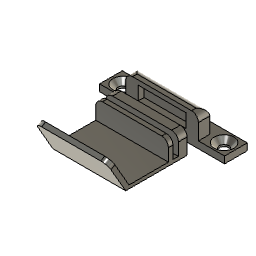
Door_Handle (Autodesk Fusion 360 design; units mm, degrees)
Autodesk Fusion 360 part; units mm, degrees
sketch "Sketch1" plane through (0, 0, 0) normal (0, 0, 1) x (1, 0, 0) in component "Door Handle"
  line L0 (16.0106, 11.1087) -> (16.0106, 8.7087)
  line L1 (-15.9894, -12.0913) -> (-15.9894, 14.9087)
  line L2 (16.0106, 8.7087) -> (16.0106, 6.7087)
  line L3 (-15.9894, 14.9087) -> (16.0106, 14.9087)
  line L4 (16.0106, 8.7087) -> (-15.9894, 8.7087)
  line L5 (16.0106, 14.9087) -> (16.0106, 11.1087)
  line L6 (16.0106, -12.0913) -> (-15.9894, -12.0913)
  line L7 (16.0106, 14.9087) -> (16.0106, -12.0913)
  line L8 (16.0106, 6.7087) -> (-15.9894, 6.7087)
  line L9 (16.0106, 11.1087) -> (-15.9894, 11.1087)
  dimension "d1" = 32
  dimension "d2" = 27
  dimension "d3" = 3.8
  dimension "d4" = 2.4
  dimension "d5" = 2
  constraint horizontal L3
  constraint vertical L7
  constraint horizontal L6
  constraint vertical L1
  constraint perpendicular L3 L5
  constraint coincident L9.end L1
  constraint perpendicular L1 L9
  constraint perpendicular L0 L9
  constraint coincident L4.end L1
  constraint perpendicular L1 L4
  constraint perpendicular L2 L4
  constraint coincident L8.end L1
  constraint perpendicular L1 L8
  measures "d1" distance of L3.end L1.end
  measures "d2" distance of L1.start L1.end
  measures "d3" distance of L3.end L0.start
  measures "d4" distance of L0.start L0.end
  measures "d5" distance of L2.end L0.end
extrude "Extrude1" add sketch "Sketch1" against normal blind 1.5 makes body 1 in component "Door Handle"
extrude "Extrude2" add sketch "Sketch1" along normal blind 8.5 contours L1 L3 L5 L7 L9 | L1 L2 L4 L7 L8 bodies 1 in component "Door Handle"
sketch "Sketch2" plane through (16.0106, 0, 0) normal (1, 0, 0) x (0, 1, 0) in component "Door Handle"
  line L0 (11.1087, 0) -> (8.7087, 0)
  line L1 (8.7087, 0) -> (8.7087, 8.5)
  line L2 (8.7087, 8.5) -> (6.7087, 8.5)
  line L3 (6.7087, 8.5) -> (6.7087, 0)
  line L4 (6.7087, 0) -> (-12.0913, 0)
  line L5 (-12.0913, 0) -> (-12.0913, -1.5)
  line L6 (-12.0913, -1.5) -> (14.9087, -1.5)
  line L7 (14.9087, -1.5) -> (14.9087, 8.5)
  line L8 (14.9087, 8.5) -> (11.1087, 8.5)
  line L9 (11.1087, 8.5) -> (11.1087, 0)
  line L10 (-12.0913, -1.5) -> (-20.0913, 12.3564)
  line L11 (-12.0913, -1.5) -> (3.9087, -1.5) construction
  line L12 (-12.0913, -1.5) -> (-10.3593, -0.5)
  line L13 (-10.3593, -0.5) -> (-18.3593, 13.3564)
  line L14 (-20.0913, 12.3564) -> (-18.3593, 13.3564)
  dimension "d10" = 120
  dimension "d11" = 16
  dimension "d12" = 2
  dimension "d13" = 16
  constraint horizontal L11
  constraint coincident L5.end L6.start
  constraint perpendicular L10 L12
  constraint perpendicular L12 L13
  measures "d10" angle of L10 L11
  measures "d11" distance of L5.end L10.end
  measures "d12" distance of L5.end L12.end
  measures "d13" distance of L12.end L13.end
extrude "Extrude3" add sketch "Sketch2" against normal blind 32 contours L4 L5 L10 L13 L14 bodies 1 in component "Door Handle"
sketch "Sketch3" plane through (0, 14.9087, 0) normal (0, 1, 0) x (-1, 0, 0) in component "Door Handle"
  line L0 (-16.0106, 8.5) -> (-16.0106, -1.5)
  line L1 (-16.0106, -1.5) -> (15.9894, -1.5)
  line L2 (15.9894, -1.5) -> (15.9894, 8.5)
  line L3 (15.9894, 8.5) -> (-16.0106, 8.5)
  circle A0 centre (-0.0106, 3.5) radius 0.5
  line L4 (-10.5106, 6.5) -> (10.4894, 6.5)
  line L5 (10.4894, 6.5) -> (10.4894, 0.5)
  line L6 (10.4894, 0.5) -> (-10.5106, 0.5)
  line L7 (-10.5106, 0.5) -> (-10.5106, 6.5)
  circle A1 centre (-0.0106, 3.5) radius 0.5
  dimension "d17" = 21
  dimension "d18" = 6
  constraint horizontal L4
  constraint vertical L5
  constraint horizontal L6
  constraint vertical L7
  constraint coincident A0.centre A1.centre
  measures "d17" distance of L4.start L4.end
  measures "d18" distance of L4.start L6.end
extrude "Extrude4" cut sketch "Sketch3" against normal blind 2.6 contours A0 A1 | L4 L5 L6 L7 bodies 1 in component "Door Handle"
fillet "Fillet1" radius 3 6 edges at (16.0106, -19.2253, 12.8564) (16.0106, 7.7087, 8.5) (16.0106, 13.0087, 8.5) (-15.9894, 13.0087, 8.5) (-15.9894, 7.7087, 8.5) (-15.9894, -19.2253, 12.8564) on bodies 1 in component "Door Handle"
sketch "Sketch1 (2)" plane through (0, 0, 0) normal (0, 0, 1) x (1, 0, 0) in component "Magnet holder"
  line L0 (-26.5987, 26.3517) -> (28.4013, 26.3517)
  line L1 (28.4013, 26.3517) -> (28.4013, 16.3517)
  line L2 (28.4013, 16.3517) -> (-26.5987, 16.3517)
  line L3 (-26.5987, 16.3517) -> (-26.5987, 26.3517)
  line L4 (-15.0987, 21.3517) -> (16.9013, 21.3517)
  line L5 (16.9013, 21.3517) -> (16.9013, 16.3517)
  line L6 (16.9013, 16.3517) -> (-15.0987, 16.3517)
  line L7 (-15.0987, 16.3517) -> (-15.0987, 21.3517)
  line L8 (-26.5987, 16.3517) -> (0.9013, 16.3517)
  line L9 (-15.0987, 16.3517) -> (0.9013, 16.3517)
  dimension "d24" = 55
  dimension "d25" = 10
  dimension "d26" = 32
  dimension "d27" = 5
  constraint horizontal L0
  constraint vertical L1
  constraint horizontal L2
  constraint vertical L3
  constraint horizontal L4
  constraint vertical L5
  constraint horizontal L6
  constraint vertical L7
  constraint midpoint L2 L8.end
  constraint midpoint L6 L8.end
  constraint coincident L8.end L9.end
  measures "d24" distance of L0.start L0.end
  measures "d25" distance of L0.start L2.end
  measures "d26" distance of L4.start L4.end
  measures "d27" distance of L4.start L6.end
extrude "Extrude1'" add sketch "Sketch1 (2)" along normal blind 13 separate body contours L2 L4 L5 L6 L7 L8 L9 makes body 2 in component "Magnet holder"
sketch "Sketch2 (2)" plane through (0, 16.3517, 0) normal (0, -1, 0) x (1, 0, 0) in component "Magnet holder"
  line L0 (-15.0987, 0) -> (16.9013, 0)
  line L1 (16.9013, 0) -> (16.9013, 13)
  line L2 (16.9013, 13) -> (-15.0987, 13)
  line L3 (-15.0987, 13) -> (-15.0987, 0)
  line L4 (-9.5987, 11) -> (11.4013, 11)
  line L5 (11.4013, 11) -> (11.4013, 5)
  line L6 (11.4013, 5) -> (-9.5987, 5)
  line L7 (-9.5987, 5) -> (-9.5987, 11)
  line L8 (-15.0987, 13) -> (-15.0987, 8)
  circle A0 centre (0.9013, 8) radius 0.5
  line L9 (-9.5987, 11) -> (11.4013, 5)
  line L10 (11.4013, 11) -> (-9.5987, 5)
  circle A1 centre (0.9013, 8) radius 0.5
  circle A2 centre (0.9013, 8) radius 0.5
  line L11 (-15.0987, 8) -> (0.9013, 8)
  dimension "d32" = 21
  dimension "d33" = 6
  dimension "d34" = 5
  dimension "d35" = 16
  dimension "d36" = 1
  dimension "d50" = 1
  dimension "d51" = 1
  constraint horizontal L4
  constraint vertical L5
  constraint horizontal L6
  constraint vertical L7
  constraint coincident L2.end L3.start
  constraint perpendicular L0 L8
  constraint midpoint L9 A0.centre
  constraint concentric A0 A2
  constraint coincident A0.centre A1.centre
  constraint perpendicular L3 L11
  measures "d32" distance of L4.start L4.end
  measures "d33" distance of L4.start L6.end
  measures "d34" distance of L2.end L8.end
  measures "d35" distance of L8.end A0.centre
  measures "d36" diameter of A0
  measures "d50" diameter of A1
  measures "d51" diameter of A2
extrude "Extrude2'" cut sketch "Sketch2 (2)" against normal blind 2.6 contours L7 A0 L9 A1 A2 L11 | L4 A0 L9 L10 A1 A2 | L5 A0 L9 L10 A1 A2 | L7 A0 L10 A1 A2 L11 | A0 L9 A1 A2 L11 | A0 L9 L10 A1 A2 | L6 A0 L9 L10 A1 A2 | A0 L9 L10 A1 A2 | A0 L10 A1 A2 L11 | A0 L9 L10 A1 A2 bodies 2 in component "Magnet holder"
extrude "Extrude3'" add sketch "Sketch1 (2)" along normal blind 3 contours L0 L1 L2 L3 L4 L5 L7 L8 bodies 2 in component "Magnet holder"
sketch "Sketch3 (2)" plane through (0, 0, 3) normal (0, 0, 1) x (-1, 0, 0) in component "Magnet holder"
  line L0 (26.5987, -26.3517) -> (26.5987, -16.3517)
  line L1 (26.5987, -16.3517) -> (15.0987, -16.3517)
  line L2 (15.0987, -16.3517) -> (15.0987, -21.3517)
  line L3 (15.0987, -21.3517) -> (-16.9013, -21.3517)
  line L4 (-16.9013, -21.3517) -> (-16.9013, -16.3517)
  line L5 (-16.9013, -16.3517) -> (-28.4013, -16.3517)
  line L6 (-28.4013, -16.3517) -> (-28.4013, -26.3517)
  line L7 (-28.4013, -26.3517) -> (26.5987, -26.3517)
  line L8 (26.5987, -21.3517) -> (21.3987, -21.3517)
  line L9 (-28.4013, -21.3517) -> (-23.2013, -21.3517)
  dimension "d41" = 5.2
  dimension "d42" = 5.2
  constraint midpoint L0 L8.start
  constraint perpendicular L0 L8
  constraint midpoint L6 L9.start
  constraint perpendicular L6 L9
  measures "d41" distance of L8.start L8.end
  measures "d42" distance of L9.start L9.end
hole "Hole1" at (23.2013, 21.3517, 3) at (-21.3987, 21.3517, 3) direction (0, 0, -1) diameter 4.2 end through all countersink diameter 8.6 countersink angle 90 bodies 2 in component "Magnet holder"
fillet "Fillet1'" radius 3 3 edges at (0.9013, 21.3517, 13) (16.9013, 18.8517, 13) (-15.0987, 18.8517, 13) on bodies 2 in component "Magnet holder"
move_body "Move1" bodies 2 to x (1, 0, 0) y (0, 1, 0) z (0, 0, 1) at (0, 5, 0) in component "Magnet holder"
component "Door Handle" placed x (1, 0, 0) y (0, 1, 0) z (0, 0, 1) at (0, 0, 0)
component "Magnet holder" placed x (1, 0, 0) y (0, 1, 0) z (0, 0, 1) at (0, 0, 0)
